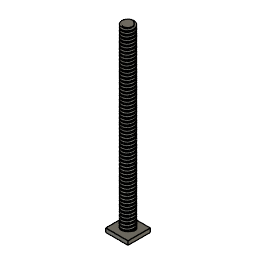
Lead Screw (Autodesk Fusion 360 design; units mm, degrees)
part number: 2026-04-26-20-37-26-178
Autodesk Fusion 360 part; units mm, degrees
sketch "Sketch3" plane through (0, 0, 0) normal (0, 0, 1) x (1, 0, 0)
  circle A0 centre (0, 0) radius 8
  dimension "d6" = 16
  constraint coincident A0.centre origin
  measures "d6" diameter of A0
extrude "Extrude2" add sketch "Sketch3" along normal blind 225
thread "Thread2" "ISO Metric Trapezoidal Threads 16.0 TR16x4 TR16x4 7e" major diameter 15.85 minor diameter 11.287 pitch 4 angle 30 modelled right hand crest width 1.4433 on face at (7.9602, -0.7965, 150) crest through (7.925, 0, -1)
sketch "Sketch5" plane through (0, 0, 0) normal (0, 0, -1) x (1, 0, 0)
  spline S0 degree 3 poles (-4.8889, 2.8191) (-5.4732, 2.3756) (-5.9613, 1.8155) (-6.7217, 0.5402) (-6.9851, -0.1687) (-7.2867, -1.7118) (-7.2993, -2.541) (-7.1796, -3.3555) knots 0 0 0 0 0.220074 0.220074 0.444076 0.444076 0.689376 0.689376 0.689376 0.689376
  arc A0 (-7.1796, -3.3555) -> (7.1796, -3.3555) centre (0, 0) ccw
  spline S1 degree 3 poles (7.1796, -3.3555) (7.3173, -2.4184) (7.2798, -1.463) (6.8745, 0.1461) (6.5911, 0.808) (5.8444, 1.9464) (5.4038, 2.4283) (4.8889, 2.8191) knots 0 0 0 0 0.284141 0.284141 0.499167 0.499167 0.694416 0.694416 0.694416 0.694416
  arc A1 (4.8889, 2.8191) -> (-4.8889, 2.8191) centre (0, 0) ccw
  line L0 (-14.25, 14.25) -> (14.25, 14.25)
  line L1 (14.25, 14.25) -> (14.25, -14.25)
  line L2 (14.25, -14.25) -> (-14.25, -14.25)
  line L3 (-14.25, -14.25) -> (-14.25, 14.25)
  line L4 (-14.25, 14.25) -> (14.25, -14.25) construction
  line L5 (14.25, 14.25) -> (-14.25, -14.25) construction
  dimension "d22" = 28.5
  dimension "d23" = 28.5
  constraint horizontal L0
  constraint perpendicular L0 L1
  constraint parallel L0 L2
  constraint parallel L1 L3
  constraint coincident L4 A0.centre
  constraint coincident L5 A0.centre
  constraint coincident A0.centre A1.centre
  measures "d22" distance of L0.end L1.end
  measures "d23" distance of L1.end L2.end
extrude "Extrude6" add sketch "Sketch5" along normal blind 5 contours S0 A0 S1 A1 | L0 L1 L2 L3
